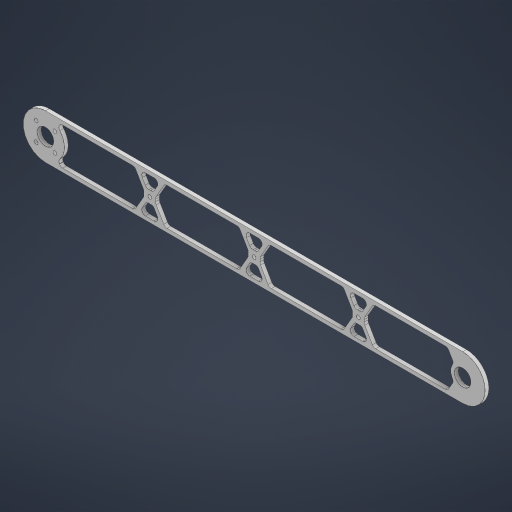
# Autodesk Inventor part: Arm3rdLinkNoServo
Saved by Autodesk Inventor 2023 (Build 270158000, 158)
## iProperties
Created: 2023-12-24
Part Number: Arm3rdLinkNoServo
Material: Generic
Document SubType Name: Modeling
Designer: kelle
Density: 1 g/cm^3
Appearance: Default
Author: kelle
Autodesk Inventor part; units mm, degrees
ref_plane "YZ Plane" through (0, 0, 0) normal (1, 0, 0) x (0, 1, 0)
ref_plane "XZ Plane" through (0, 0, 0) normal (0, 1, 0) x (-1, 0, 0)
ref_plane "XY Plane" through (0, 0, 0) normal (0, 0, 1) x (1, 0, 0)
sketch "Sketch1" plane through (0, 0, 0) normal (0, 0, 1) x (1, 0, 0)
  line L0 (-177.8, 0) -> (177.8, 0) construction
  line L1 (-177.8, -19.05) -> (177.8, -19.05)
  line L2 (177.8, 19.05) -> (-177.8, 19.05)
  arc A0 (-177.8, 19.05) -> (-177.8, -19.05) centre (-177.8, 0) ccw
  arc A1 (177.8, -19.05) -> (177.8, 19.05) centre (177.8, 0) ccw
  line L3 (-185.8, -8) -> (-169.8, -8) construction
  line L4 (-169.8, -8) -> (-169.8, 8) construction
  line L5 (-169.8, 8) -> (-185.8, 8) construction
  line L6 (-185.8, 8) -> (-185.8, -8) construction
  line L7 (-185.8, -8) -> (-169.8, 8) construction
  line L8 (-169.8, -8) -> (-185.8, 8) construction
  circle A2 centre (-185.8, 8) radius 1.5875
  circle A3 centre (-169.8, 8) radius 1.5875
  circle A4 centre (-185.8, -8) radius 1.5875
  circle A5 centre (-169.8, -8) radius 1.5875
  circle A6 centre (-177.8, 0) radius 7
  circle A7 centre (177.8, 0) radius 7
  circle A8 centre (0, 0) radius 2
  circle A9 centre (88.9, 0) radius 2
  circle A10 centre (-88.9, 0) radius 2
  circle A11 centre (0, 0) radius 2
  dimension "d0" = 177.8
  dimension "d1" = 38.1
  dimension "d3" = 16
  dimension "d4" = 16
  dimension "d5" = 3.175
  dimension "d8" = 16
  dimension "d11" = 16
  dimension "d14" = 14
  dimension "d15" = 14
  dimension "d16" = 4
  dimension "d19" = 88.9
  dimension "d22" = 88.9
  constraints: 20 end point, 12 centre point, 7 coincident, 4 horizontal, 4 point on circle, 4 tangent, 3 midpoint, 3 parallel, 1 perpendicular, 1 vertical, 15 other
  measures "d0" distance of point (0, 0) L0.end
  measures "d1" diameter of A1
  measures "d3" distance of L3.start L3.end
  measures "d4" distance of L4.end L3.end
  measures "d5" diameter of A2
  measures "d8" distance of A2.centre A3.centre
  measures "d11" distance of A2.centre A4.centre
  measures "d14" diameter of A6
  measures "d15" diameter of A7
  measures "d16" diameter of A8
  measures "d19" distance of point (0, 0) point (88.9, 0)
  measures "d22" distance of point (0, 0) point (-88.9, 0)
extrude "Extrusion1" add sketch "Sketch1" along normal blind 3.175
sketch "Sketch4" plane through (0, 0, 3.175) normal (0, 0, 1) x (1, 0, 0)
  arc A0 (177.8, -19.05) -> (177.8, 19.05) centre (177.8, 0) ccw projected
  line L0 (177.8, 19.05) -> (-177.8, 19.05) projected
  arc A1 (-177.8, 19.05) -> (-177.8, -19.05) centre (-177.8, 0) ccw projected
  line L1 (-177.8, -19.05) -> (177.8, -19.05) projected
  circle A2 centre (0, 0) radius 2 projected
  circle A3 centre (88.9, 0) radius 2 projected
  circle A4 centre (-88.9, 0) radius 2 projected
  circle A5 centre (177.8, 0) radius 7 projected
  circle A6 centre (-177.8, 0) radius 7 projected
  circle A7 centre (-169.8, -8) radius 1.5875 projected
  circle A8 centre (-185.8, -8) radius 1.5875 projected
  circle A9 centre (-169.8, 8) radius 1.5875 projected
  circle A10 centre (-185.8, 8) radius 1.5875 projected
  line L2 (-177.8, 15.875) -> (177.8, 15.875)
  arc A11 (177.8, -15.875) -> (177.8, 15.875) centre (177.8, 0) ccw
  line L3 (177.8, -15.875) -> (-177.8, -15.875)
  arc A12 (-177.8, 15.875) -> (-177.8, -15.875) centre (-177.8, 0) ccw
  circle A13 centre (-177.8, 0) radius 7 construction
  circle A14 centre (-177.8, 0) radius 12.9012 construction
  circle A15 centre (-177.8, 0) radius 16.0762
  circle A16 centre (177.8, 0) radius 10.175
  circle A17 centre (88.9, 0) radius 5.175
  circle A18 centre (0, 0) radius 5.175
  circle A19 centre (-88.9, 0) radius 5.175
  circle A20 centre (-88.9, 0) radius 2 construction
  line L4 (-177.8, 0) -> (-88.9, 0) construction
  line L5 (-177.8, 0) -> (-155.575, 38.4948)
  line L6 (-155.575, 38.4948) -> (-111.125, 38.4948)
  line L7 (-111.125, 38.4948) -> (-88.9, 0)
  line L8 (-88.9, 0) -> (-111.125, -38.4948)
  line L9 (-111.125, -38.4948) -> (-155.575, -38.4948)
  line L10 (-155.575, -38.4948) -> (-177.8, 0)
  line L11 (-92.5662, 0) -> (-112.9581, 35.3198)
  line L12 (-112.9581, 35.3198) -> (-153.7419, 35.3198)
  line L13 (-153.7419, 35.3198) -> (-174.1338, 0)
  line L14 (-174.1338, 0) -> (-153.7419, -35.3198)
  line L15 (-153.7419, -35.3198) -> (-112.9581, -35.3198)
  line L16 (-112.9581, -35.3198) -> (-92.5662, 0)
  line L17 (-88.9, 19.05) -> (-88.9, -19.05) construction
  line L18 (0, 19.05) -> (0, -19.05) construction
  line L19 (0, 0) -> (-22.225, 38.4948)
  line L20 (-66.675, 38.4948) -> (-88.9, 0)
  line L21 (-88.9, 0) -> (-66.675, -38.4948)
  line L22 (-22.225, -38.4948) -> (0, 0)
  line L23 (-85.2338, 0) -> (-64.8419, 35.3198)
  line L24 (-24.0581, 35.3198) -> (-3.6662, 0)
  line L25 (-3.6662, 0) -> (-24.0581, -35.3198)
  line L26 (-64.8419, -35.3198) -> (-85.2338, 0)
  line L27 (177.8, 0) -> (155.575, 38.4948)
  line L28 (111.125, 38.4948) -> (88.9, 0)
  line L29 (88.9, 0) -> (111.125, -38.4948)
  line L30 (155.575, -38.4948) -> (177.8, 0)
  line L31 (92.5662, 0) -> (112.9581, 35.3198)
  line L32 (153.7419, 35.3198) -> (174.1338, 0)
  line L33 (174.1338, 0) -> (153.7419, -35.3198)
  line L34 (112.9581, -35.3198) -> (92.5662, 0)
  line L35 (66.675, 38.4948) -> (88.9, 0)
  line L36 (85.2338, 0) -> (64.8419, 35.3198)
  line L37 (24.0581, 35.3198) -> (3.6662, 0)
  line L38 (0, 0) -> (22.225, 38.4948)
  line L39 (3.6662, 0) -> (24.0581, -35.3198)
  line L40 (22.225, -38.4948) -> (0, 0)
  line L41 (64.8419, -35.3198) -> (85.2338, 0)
  line L42 (88.9, 0) -> (66.675, -38.4948)
  point P0 (-133.35, 0)
  point P1 (79.7346, 15.875)
  point P2 (86.3125, 4.4817)
  point P3 (91.4875, 4.4817)
  point P4 (98.0654, 15.875)
  point P5 (86.3125, -4.4817)
  point P6 (79.7346, -15.875)
  point P7 (98.0654, -15.875)
  point P8 (91.4875, -4.4817)
  point P9 (9.1654, -15.875)
  point P10 (2.5875, -4.4817)
  point P11 (-2.5875, -4.4817)
  point P12 (-9.1654, -15.875)
  point P13 (2.5875, 4.4817)
  point P14 (9.1654, 15.875)
  point P15 (-9.1654, 15.875)
  point P16 (-2.5875, 4.4817)
  point P17 (-86.3125, 4.4817)
  point P18 (-79.7346, 15.875)
  point P19 (-98.0654, 15.875)
  point P20 (-91.4875, 4.4817)
  point P21 (-79.7346, -15.875)
  point P22 (-86.3125, -4.4817)
  point P23 (-91.4875, -4.4817)
  point P24 (-98.0654, -15.875)
  point P25 (93.6929, -1.9516)
  point P26 (101.7316, -15.875)
  point P27 (164.9684, -15.875)
  point P28 (170.2169, -6.7843)
  point P29 (170.2169, 6.7843)
  point P30 (164.9684, 15.875)
  point P31 (101.7316, 15.875)
  point P32 (93.6929, 1.9516)
  point P33 (4.7929, -1.9516)
  point P34 (12.8316, -15.875)
  point P35 (76.0684, -15.875)
  point P36 (84.1071, -1.9516)
  point P37 (84.1071, 1.9516)
  point P38 (76.0684, 15.875)
  point P39 (12.8316, 15.875)
  point P40 (4.7929, 1.9516)
  point P41 (-84.1071, -1.9516)
  point P42 (-76.0684, -15.875)
  point P43 (-12.8316, -15.875)
  point P44 (-4.7929, -1.9516)
  point P45 (-4.7929, 1.9516)
  point P46 (-12.8316, 15.875)
  point P47 (-76.0684, 15.875)
  point P48 (-84.1071, 1.9516)
  point P49 (-101.7316, -15.875)
  point P50 (-93.6929, -1.9516)
  point P51 (-93.6929, 1.9516)
  point P52 (-101.7316, 15.875)
  point P53 (-164.9684, 15.875)
  point P54 (-167.1706, 12.0607)
  point P55 (-167.1706, -12.0607)
  point P56 (-164.9684, -15.875)
  dimension "d54" = 3.175
  dimension "d55" = 3.175
  dimension "d56" = 3.175
  dimension "d57" = 3.175
  dimension "d58" = 3.175
  dimension "d59" = 3.175
  dimension "d60" = 3.175
  constraints: 82 end point, 33 symmetric about line, 8 centre point, 4 point on circle, 3 midpoint, 2 point on line, 1 coincident, 1 perpendicular, 1 tangent, 21 other
  measures "d54" distance between parallel lines of L0 L2
  measures "d55" radial gap between concentric circles of A14 A15
  measures "d56" radial gap between concentric circles of A5 A16
  measures "d57" radial gap between concentric circles of A3 A17
  measures "d58" radial gap between concentric circles of A2 A18
  measures "d59" radial gap between concentric circles of A4 A19
  measures "d60" distance between parallel lines of L7 L11
extrude "Extrusion4" cut sketch "Sketch4" against normal through all contours L3 L34 A17 L31 L2 L32 A16 L33 | L3 L42 A17 L29 | L28 A17 L35 L2 | L3 L39 A18 L37 L2 L36 A17 L41 | L3 L22 A18 L40 | L38 A18 L19 L2 | L3 L26 A19 L23 L2 L24 A18 L25 | L3 L8 A19 L21 | L20 A19 L7 L2 | L3 L14 A15 L13 L2 L11 A19 L16
fillet "Fillet2" radius 3.175 56 edges at (-86.3125, -4.4817, 1.5875) (-79.7346, -15.875, 1.5875) (-91.4875, -4.4817, 1.5875) (-98.0654, -15.875, 1.5875) (-93.6929, -1.9516, 1.5875) (-101.7316, -15.875, 1.5875) (-93.6929, 1.9516, 1.5875) (-101.7316, 15.875, 1.5875) (-164.9684, 15.875, 1.5875) (-167.1706, 12.0607, 1.5875) (-167.1706, -12.0607, 1.5875) (-164.9684, -15.875, 1.5875) (-76.0684, -15.875, 1.5875) (-84.1071, -1.9516, 1.5875) (-12.8316, -15.875, 1.5875) (-4.7929, -1.9516, 1.5875) (-4.7929, 1.9516, 1.5875) (-12.8316, 15.875, 1.5875) (-76.0684, 15.875, 1.5875) (-84.1071, 1.9516, 1.5875) (2.5875, -4.4817, 1.5875) (9.1654, -15.875, 1.5875) (-2.5875, -4.4817, 1.5875) (-9.1654, -15.875, 1.5875) (79.7346, -15.875, 1.5875) (86.3125, -4.4817, 1.5875) (98.0654, -15.875, 1.5875) (91.4875, -4.4817, 1.5875) (12.8316, -15.875, 1.5875) (4.7929, -1.9516, 1.5875) (76.0684, -15.875, 1.5875) (84.1071, -1.9516, 1.5875) (84.1071, 1.9516, 1.5875) (76.0684, 15.875, 1.5875) (12.8316, 15.875, 1.5875) (4.7929, 1.9516, 1.5875) (-79.7346, 15.875, 1.5875) (-86.3125, 4.4817, 1.5875) (-98.0654, 15.875, 1.5875) (-91.4875, 4.4817, 1.5875) (101.7316, -15.875, 1.5875) (93.6929, -1.9516, 1.5875) (164.9684, -15.875, 1.5875) (170.2169, -6.7843, 1.5875) (170.2169, 6.7843, 1.5875) (164.9684, 15.875, 1.5875) (101.7316, 15.875, 1.5875) (93.6929, 1.9516, 1.5875) (9.1654, 15.875, 1.5875) (2.5875, 4.4817, 1.5875) (-9.1654, 15.875, 1.5875) (-2.5875, 4.4817, 1.5875) (86.3125, 4.4817, 1.5875) (79.7346, 15.875, 1.5875) (91.4875, 4.4817, 1.5875) (98.0654, 15.875, 1.5875)
sketch "Sketch5" plane through (0, 0, 3.175) normal (0, 0, 1) x (1, 0, 0)
  line L0 (83.4393, -3.1082) -> (76.9849, -14.2875) projected
  arc A0 (74.2353, -15.875) -> (76.9849, -14.2875) centre (74.2353, -12.7) ccw projected
  line L1 (74.2353, -15.875) -> (14.6647, -15.875) projected
  arc A1 (11.9151, -14.2875) -> (14.6647, -15.875) centre (14.6647, -12.7) ccw projected
  line L2 (11.9151, -14.2875) -> (5.4607, -3.1082) projected
  arc A2 (5.0885, -0.9425) -> (5.4607, -3.1082) centre (8.2103, -1.5207) ccw projected
  arc A3 (5.0885, -0.9425) -> (5.0885, 0.9425) centre (0, 0) ccw projected
  arc A4 (5.4607, 3.1082) -> (5.0885, 0.9425) centre (8.2103, 1.5207) ccw projected
  line L3 (5.4607, 3.1082) -> (11.9151, 14.2875) projected
  arc A5 (14.6647, 15.875) -> (11.9151, 14.2875) centre (14.6647, 12.7) ccw projected
  line L4 (14.6647, 15.875) -> (74.2353, 15.875) projected
  arc A6 (76.9849, 14.2875) -> (74.2353, 15.875) centre (74.2353, 12.7) ccw projected
  line L5 (76.9849, 14.2875) -> (83.4393, 3.1082) projected
  arc A7 (83.8115, 0.9425) -> (83.4393, 3.1082) centre (80.6897, 1.5207) ccw projected
  arc A8 (83.8115, 0.9425) -> (83.8115, -0.9425) centre (88.9, 0) ccw projected
  arc A9 (83.4393, -3.1082) -> (83.8115, -0.9425) centre (80.6897, -1.5207) ccw projected
  line L6 (-3.8614, 6.6882) -> (-6.4158, 11.1125) projected
  arc A10 (-3.6662, 15.875) -> (-6.4158, 11.1125) centre (-3.6662, 12.7) ccw projected
  line L7 (-3.6662, 15.875) -> (3.6662, 15.875) projected
  arc A11 (6.4158, 11.1125) -> (3.6662, 15.875) centre (3.6662, 12.7) ccw projected
  line L8 (6.4158, 11.1125) -> (3.8614, 6.6882) projected
  arc A12 (0.689, 5.1289) -> (3.8614, 6.6882) centre (1.1118, 8.2757) ccw projected
  arc A13 (0.689, 5.1289) -> (-0.689, 5.1289) centre (0, 0) ccw projected
  arc A14 (-3.8614, 6.6882) -> (-0.689, 5.1289) centre (-1.1118, 8.2757) ccw projected
  line L9 (95.3158, 11.1125) -> (92.7614, 6.6882) projected
  arc A15 (89.589, 5.1289) -> (92.7614, 6.6882) centre (90.0118, 8.2757) ccw projected
  arc A16 (89.589, 5.1289) -> (88.211, 5.1289) centre (88.9, 0) ccw projected
  arc A17 (85.0386, 6.6882) -> (88.211, 5.1289) centre (87.7882, 8.2757) ccw projected
  line L10 (85.0386, 6.6882) -> (82.4842, 11.1125) projected
  arc A18 (85.2338, 15.875) -> (82.4842, 11.1125) centre (85.2338, 12.7) ccw projected
  line L11 (85.2338, 15.875) -> (92.5662, 15.875) projected
  arc A19 (95.3158, 11.1125) -> (92.5662, 15.875) centre (92.5662, 12.7) ccw projected
  line L12 (-92.7614, 6.6882) -> (-95.3158, 11.1125) projected
  arc A20 (-92.5662, 15.875) -> (-95.3158, 11.1125) centre (-92.5662, 12.7) ccw projected
  line L13 (-92.5662, 15.875) -> (-85.2338, 15.875) projected
  arc A21 (-82.4842, 11.1125) -> (-85.2338, 15.875) centre (-85.2338, 12.7) ccw projected
  line L14 (-82.4842, 11.1125) -> (-85.0386, 6.6882) projected
  arc A22 (-88.211, 5.1289) -> (-85.0386, 6.6882) centre (-87.7882, 8.2757) ccw projected
  arc A23 (-88.211, 5.1289) -> (-89.589, 5.1289) centre (-88.9, 0) ccw projected
  arc A24 (-92.7614, 6.6882) -> (-89.589, 5.1289) centre (-90.0118, 8.2757) ccw projected
  line L15 (-5.4607, -3.1082) -> (-11.9151, -14.2875) projected
  arc A25 (-14.6647, -15.875) -> (-11.9151, -14.2875) centre (-14.6647, -12.7) ccw projected
  line L16 (-14.6647, -15.875) -> (-74.2353, -15.875) projected
  arc A26 (-76.9849, -14.2875) -> (-74.2353, -15.875) centre (-74.2353, -12.7) ccw projected
  line L17 (-76.9849, -14.2875) -> (-83.4393, -3.1082) projected
  arc A27 (-83.8115, -0.9425) -> (-83.4393, -3.1082) centre (-80.6897, -1.5207) ccw projected
  arc A28 (-83.8115, -0.9425) -> (-83.8115, 0.9425) centre (-88.9, 0) ccw projected
  arc A29 (-83.4393, 3.1082) -> (-83.8115, 0.9425) centre (-80.6897, 1.5207) ccw projected
  line L18 (-83.4393, 3.1082) -> (-76.9849, 14.2875) projected
  arc A30 (-74.2353, 15.875) -> (-76.9849, 14.2875) centre (-74.2353, 12.7) ccw projected
  line L19 (-74.2353, 15.875) -> (-14.6647, 15.875) projected
  arc A31 (-11.9151, 14.2875) -> (-14.6647, 15.875) centre (-14.6647, 12.7) ccw projected
  line L20 (-11.9151, 14.2875) -> (-5.4607, 3.1082) projected
  arc A32 (-5.0885, 0.9425) -> (-5.4607, 3.1082) centre (-8.2103, 1.5207) ccw projected
  arc A33 (-5.0885, 0.9425) -> (-5.0885, -0.9425) centre (0, 0) ccw projected
  arc A34 (-5.4607, -3.1082) -> (-5.0885, -0.9425) centre (-8.2103, -1.5207) ccw projected
  line L21 (169.1788, -8.5823) -> (165.8849, -14.2875) projected
  arc A35 (163.1353, -15.875) -> (165.8849, -14.2875) centre (163.1353, -12.7) ccw projected
  line L22 (163.1353, -15.875) -> (103.5647, -15.875) projected
  arc A36 (100.8151, -14.2875) -> (103.5647, -15.875) centre (103.5647, -12.7) ccw projected
  line L23 (100.8151, -14.2875) -> (94.3607, -3.1082) projected
  arc A37 (93.9885, -0.9425) -> (94.3607, -3.1082) centre (97.1103, -1.5207) ccw projected
  arc A38 (93.9885, -0.9425) -> (93.9885, 0.9425) centre (88.9, 0) ccw projected
  arc A39 (94.3607, 3.1082) -> (93.9885, 0.9425) centre (97.1103, 1.5207) ccw projected
  line L24 (94.3607, 3.1082) -> (100.8151, 14.2875) projected
  arc A40 (103.5647, 15.875) -> (100.8151, 14.2875) centre (103.5647, 12.7) ccw projected
  line L25 (103.5647, 15.875) -> (163.1353, 15.875) projected
  arc A41 (165.8849, 14.2875) -> (163.1353, 15.875) centre (163.1353, 12.7) ccw projected
  line L26 (165.8849, 14.2875) -> (169.1788, 8.5823) projected
  arc A42 (169.1335, 5.3312) -> (169.1788, 8.5823) centre (166.4292, 6.9948) ccw projected
  arc A43 (169.1335, 5.3312) -> (169.1335, -5.3312) centre (177.8, 0) ccw projected
  arc A44 (169.1788, -8.5823) -> (169.1335, -5.3312) centre (166.4292, -6.9948) ccw projected
  line L27 (-6.4158, -11.1125) -> (-3.8614, -6.6882) projected
  arc A45 (-0.689, -5.1289) -> (-3.8614, -6.6882) centre (-1.1118, -8.2757) ccw projected
  arc A46 (-0.689, -5.1289) -> (0.689, -5.1289) centre (0, 0) ccw projected
  arc A47 (3.8614, -6.6882) -> (0.689, -5.1289) centre (1.1118, -8.2757) ccw projected
  line L28 (3.8614, -6.6882) -> (6.4158, -11.1125) projected
  arc A48 (3.6662, -15.875) -> (6.4158, -11.1125) centre (3.6662, -12.7) ccw projected
  line L29 (3.6662, -15.875) -> (-3.6662, -15.875) projected
  arc A49 (-6.4158, -11.1125) -> (-3.6662, -15.875) centre (-3.6662, -12.7) ccw projected
  line L30 (92.7614, -6.6882) -> (95.3158, -11.1125) projected
  arc A50 (92.5662, -15.875) -> (95.3158, -11.1125) centre (92.5662, -12.7) ccw projected
  line L31 (92.5662, -15.875) -> (85.2338, -15.875) projected
  arc A51 (82.4842, -11.1125) -> (85.2338, -15.875) centre (85.2338, -12.7) ccw projected
  line L32 (82.4842, -11.1125) -> (85.0386, -6.6882) projected
  arc A52 (88.211, -5.1289) -> (85.0386, -6.6882) centre (87.7882, -8.2757) ccw projected
  arc A53 (88.211, -5.1289) -> (89.589, -5.1289) centre (88.9, 0) ccw projected
  arc A54 (92.7614, -6.6882) -> (89.589, -5.1289) centre (90.0118, -8.2757) ccw projected
  line L33 (-95.3158, -11.1125) -> (-92.7614, -6.6882) projected
  arc A55 (-89.589, -5.1289) -> (-92.7614, -6.6882) centre (-90.0118, -8.2757) ccw projected
  arc A56 (-89.589, -5.1289) -> (-88.211, -5.1289) centre (-88.9, 0) ccw projected
  arc A57 (-85.0386, -6.6882) -> (-88.211, -5.1289) centre (-87.7882, -8.2757) ccw projected
  line L34 (-85.0386, -6.6882) -> (-82.4842, -11.1125) projected
  arc A58 (-85.2338, -15.875) -> (-82.4842, -11.1125) centre (-85.2338, -12.7) ccw projected
  line L35 (-85.2338, -15.875) -> (-92.5662, -15.875) projected
  arc A59 (-95.3158, -11.1125) -> (-92.5662, -15.875) centre (-92.5662, -12.7) ccw projected
  line L36 (-100.8151, 14.2875) -> (-94.3607, 3.1082) projected
  arc A60 (-93.9885, 0.9425) -> (-94.3607, 3.1082) centre (-97.1103, 1.5207) ccw projected
  arc A61 (-93.9885, 0.9425) -> (-93.9885, -0.9425) centre (-88.9, 0) ccw projected
  arc A62 (-94.3607, -3.1082) -> (-93.9885, -0.9425) centre (-97.1103, -1.5207) ccw projected
  line L37 (-94.3607, -3.1082) -> (-100.8151, -14.2875) projected
  arc A63 (-103.5647, -15.875) -> (-100.8151, -14.2875) centre (-103.5647, -12.7) ccw projected
  line L38 (-103.5647, -15.875) -> (-163.1353, -15.875) projected
  arc A64 (-165.8849, -14.2875) -> (-163.1353, -15.875) centre (-163.1353, -12.7) ccw projected
  line L39 (-165.8849, -14.2875) -> (-165.9635, -14.1515) projected
  arc A65 (-165.6195, -10.4919) -> (-165.9635, -14.1515) centre (-163.2138, -12.564) ccw projected
  arc A66 (-165.6195, -10.4919) -> (-165.6195, 10.4919) centre (-177.8, 0) ccw projected
  arc A67 (-165.9635, 14.1515) -> (-165.6195, 10.4919) centre (-163.2138, 12.564) ccw projected
  line L40 (-165.9635, 14.1515) -> (-165.8849, 14.2875) projected
  arc A68 (-163.1353, 15.875) -> (-165.8849, 14.2875) centre (-163.1353, 12.7) ccw projected
  line L41 (-163.1353, 15.875) -> (-103.5647, 15.875) projected
  arc A69 (-100.8151, 14.2875) -> (-103.5647, 15.875) centre (-103.5647, 12.7) ccw projected
  arc A70 (177.8, -19.05) -> (177.8, 19.05) centre (177.8, 0) ccw projected
  line L42 (177.8, 19.05) -> (-177.8, 19.05) projected
  arc A71 (-177.8, 19.05) -> (-177.8, -19.05) centre (-177.8, 0) ccw projected
  line L43 (-177.8, -19.05) -> (177.8, -19.05) projected
  circle A72 centre (0, 0) radius 2 projected
  circle A73 centre (88.9, 0) radius 2 projected
  circle A74 centre (-88.9, 0) radius 2 projected
  circle A75 centre (177.8, 0) radius 7 projected
  circle A76 centre (-177.8, 0) radius 7 projected
  circle A77 centre (-169.8, -8) radius 1.5875 projected
  circle A78 centre (-185.8, -8) radius 1.5875 projected
  circle A79 centre (-169.8, 8) radius 1.5875 projected
  circle A80 centre (-185.8, 8) radius 1.5875 projected
  circle A81 centre (-88.9, 0) radius 1.5875
  circle A82 centre (0, 0) radius 2 projected
  circle A83 centre (0, 0) radius 1.5875
  circle A84 centre (88.9, 0) radius 2 projected
  circle A85 centre (88.9, 0) radius 1.5875
  dimension "d64" = 3.175
  dimension "d65" = 3.175
  dimension "d66" = 3.175
  constraints: 3 centre point, 3 coincident
  measures "d64" diameter of A81
  measures "d65" diameter of A83
  measures "d66" diameter of A85
extrude "Extrusion5" add sketch "Sketch5" against normal blind 3.175 contours A72 | A73 | A74
body "Solid1"
